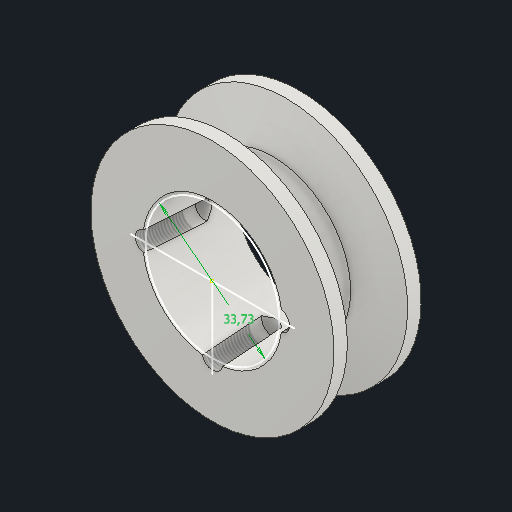
# Autodesk Inventor part: Poulie à gorge2
Saved by Autodesk Inventor 2026.2 (Build 302298010, 298A)
## iProperties
CustomPartVersion: 1
Created: 2026-03-31
Part Number: Poulie à gorge2
Material: Steel
Document SubType Name: Modeling
Designer: romai
Density: 1 g/cm^3
Appearance: Steel
Author: romai
Autodesk Inventor part; units mm, degrees
ref_plane "YZ Plane" through (0, 0, 0) normal (1, 0, 0) x (0, 1, 0)
ref_plane "XZ Plane" through (0, 0, 0) normal (0, 1, 0) x (-1, 0, 0)
sketch "Esquisse principale" plane through (0, 0, 0) normal (1, 0, 0) x (0, 1, 0)
  line L0 (0, 22) -> (30.65, 22)
  line L1 (30.65, 22) -> (30.65, 18.6115)
  line L2 (30.65, 18.6115) -> (19.65, 15.2484)
  line L3 (19.65, 15.2484) -> (19.65, 6.7516)
  line L4 (19.65, 6.7516) -> (30.65, 3.3885)
  line L5 (30.65, 3.3885) -> (30.65, 0)
  line L6 (30.65, 0) -> (0, 0)
  line L7 (28.65, 18) -> (28.65, 4) construction
  line L8 (19.65, 11) -> (28.65, 11) construction
  line L9 (30.65, 18.6115) -> (30.65, 3.3885)
  line L10 (0, -4.4) -> (0, 26.4) projected
  line L11 (0, 0) -> (0, 22)
  dimension "d0" = 14
  dimension "d1" = 34
  dimension "d2" = 2
  dimension "d6" = 22
  dimension "d21" = 57.3
  dimension "d25" = 11
  dimension "d27" = 11
  constraints: 22 end point, 5 perpendicular, 2 collinear, 2 midpoint, 2 point on line, 1 parallel
  measures "d0" distance of L7.start L7.end
  measures "d1" angle of L2 L4
  measures "d2" distance between parallel lines of L1 L7
  measures "d6" distance between parallel lines of L6 L0
  measures "d21" diameter of L7 L10
  measures "d25" distance between parallel lines of L3 L9
  measures "d27" distance between parallel lines of L6 L8
ref_plane "Plan de courroie" through (0, 19.65, 11) normal (0, 0, 1) x (1, 0, 0)
revolve "Corps" add sketch "Esquisse principale" angle 360 about axis through (0, 0, -10) along (0, 0, 1)
revolve "Bord" cut sketch "Esquisse principale" angle 360 about axis through (0, 0, -10) along (0, 0, 1) contours L9 L4 L3 L2
fillet "Congé externe" [suppressed]
fillet "Congé interne" [suppressed]
pattern_of_one "Réseau de bords"
sketch "Esquisse5" plane through (0, 0, 0) normal (1, 0, 0) x (0, 1, 0)
  line L0 (0, -3.4128) -> (0, 36.612)
  line L1 (-30.65, 22) -> (30.65, 22) projected
  line L2 (0, 22.15) -> (17.6, 22.15)
  line L3 (0, -0.15) -> (16, -0.15)
  line L4 (16, -0.15) -> (17.6, 22.15)
  line L5 (-30.65, 0) -> (30.65, 0) projected
  point P0 (0, 0)
  point P1 (0, 0)
  point P2 (16.0108, 0)
  point P3 (17.5892, 22)
  point P4 (0, 22)
  dimension "d42" = 17.6
  dimension "d43" = 16
  dimension "d44" = 22.3
  dimension "d45" = 0.15
  constraints: 8 end point, 2 horizontal, 2 point on line, 1 vertical
  measures "d42" distance of L2.start L2.end
  measures "d43" distance of L3.start L3.end
  measures "d44" distance between parallel lines of L3 L2
  measures "d45" distance between parallel lines of L5 L3
revolve "Révolution4" cut sketch "Esquisse5" angle 360 about axis through (0, 0, -3.4128) along (0, 0, 1) contours L0 L1 L4 L5
sketch "Esquisse6" plane through (0, 0, 22) normal (0, 0, 1) x (1, 0, 0)
  circle A0 centre (0, 0) radius 16.865
  line L0 (0, 0) -> (0, -20.3101)
  line L1 (0, 0) -> (20.7504, 0)
  line L2 (0, 0) -> (-20.5452, 0)
  point P0 (0, -16.865)
  point P1 (-16.865, 0)
  point P2 (16.865, 0)
  dimension "d54" = 33.73
  constraints: 6 end point, 3 point on circle, 3 point on line, 2 horizontal, 1 centre point, 1 coincident, 1 vertical
  measures "d54" diameter of A0
hole "Perçage2" at (0, -16.865, 22) at (-16.865, 0, 22) at (16.865, 0, 22) direction (0, 0, -1) diameter 5.1881 depth 15 tip angle 118 thread size "M6x0.75" class "6H" standard "ANSI Metric M Profile"
equation "\"d0\" = da_Bw"
equation "\"d1\" = da_Alfa"
equation "\"d2\" = da_c"
equation "\"d21\" = da_Dw"
equation "\"d25\" = da_Hd"
equation "\"d27\" = da_Se"
equation "\"da_r1\" = 0"
equation "\"da_r2\" = 0"
equation "\"d18\" = da_Sg"
equation "\"d5\" = da_Se"
equation "\"da_Bw\" = 14"
equation "\"da_Alfa\" = 34deg"
equation "\"da_c\" = 2"
equation "\"da_Dw\" = 57.3"
equation "\"da_Hd\" = 11"
equation "\"da_Se\" = 11"
equation "\"da_Sg\" = 12"
body "Solid1"
